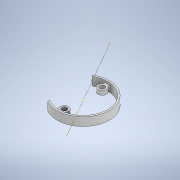
# Autodesk Inventor part: Parachute_Verb
Saved by Autodesk Inventor 2020 (Build 240168000, 168)
## iProperties
Created: 2022-04-20
Part Number: Parachute_Verb
Material: Generisch
Document SubType Name: Modeling
Designer: sp
Density: 1 g/cm^3
Appearance: Vorgabe
Author: sp
Autodesk Inventor part; units mm, degrees
ref_plane "YZ Plane" through (0, 0, 0) normal (1, 0, 0) x (0, 1, 0)
ref_plane "XZ Plane" through (0, 0, 0) normal (0, 1, 0) x (-1, 0, 0)
ref_plane "XY Plane" through (0, 0, 0) normal (0, 0, 1) x (1, 0, 0)
sketch "Skizze1" plane through (0, 0, 0) normal (0, 1, 0) x (-1, 0, 0)
  circle A0 centre (0, 0) radius 29
  circle A1 centre (0, 0) radius 31
  dimension "d0" = 58
  dimension "d1" = 62
  constraints: 2 centre point, 2 coincident
  measures "d0" diameter of A0
  measures "d1" diameter of A1
extrude "Extrusion1" add sketch "Skizze1" along normal mid plane 10
sketch "Skizze2" plane through (0, 0, 0) normal (0, 1, 0) x (-1, 0, 0)
  circle A0 centre (0, 22.5) radius 3
  circle A1 centre (0, -22.5) radius 3
  line L0 (44.9262, 0) -> (-43.1306, 0) construction
  circle A2 centre (0, -22.5) radius 5
  circle A3 centre (0, 22.5) radius 5
  line L1 (0, 38.6377) -> (0, -60.2779) construction
  line L2 (3, 30.0945) -> (-3, 30.0945)
  line L3 (-3, 30.0945) -> (-3, -30.0165)
  line L4 (-3, -30.0165) -> (3, -30.0165)
  line L5 (3, -30.0165) -> (3, 30.0945)
  point P0 (0, 0)
  point P1 (-3, 26.5)
  point P2 (3, 26.5)
  point P3 (-3, -26.5)
  point P4 (3, -26.5)
  dimension "d4" = 45
  dimension "d5" = 6
  dimension "d6" = 6
  dimension "d7" = 10
  dimension "d8" = 10
  dimension "d9" = 6
  constraints: 12 end point, 4 centre point, 2 coincident, 2 horizontal, 2 parallel, 2 point on line, 1 perpendicular, 1 symmetric about line, 1 vertical, 1 other
  measures "d4" distance of A1.centre A0.centre
  measures "d5" diameter of A1
  measures "d6" diameter of A0
  measures "d7" diameter of A3
  measures "d8" diameter of A2
  measures "d9" distance between parallel lines of L3 L5
extrude "Extrusion2" add sketch "Skizze2" along normal mid plane 5 contours L5 A3 L3 A0 | L5 A3 | A0 L3 A3 L5 | L3 A3 | A3 L3 L2 L5 | L5 A1 L3 A2 | A2 L5 | L3 A2 | L5 A2 L3 A1 | A2 L5 L4 L3
sketch "Skizze3" plane through (0, 0, 0) normal (0, 1, 0) x (-1, 0, 0)
  line L0 (-33.7018, 58.3732) -> (42.9469, -74.3862) construction
  line L1 (43.8309, 75.9173) -> (-26.6916, -46.2313) construction
  line L2 (0, 58.0617) -> (0, -82.342) construction
  circle A0 centre (0, 0) radius 31
  circle A1 centre (0, 0) radius 29
  line L3 (17.8979, 31) -> (12.398, 21.474)
  line L4 (13.0797, -22.6548) -> (20.1593, -34.9169)
  point P0 (14.5, -25.1147)
  point P1 (15.5, -26.8468)
  point P2 (15.5, 26.8468)
  point P3 (14.5, 25.1147)
  dimension "d12" = 120
  dimension "d13" = 30
  constraints: 10 end point, 7 point on line, 3 coincident, 2 centre point, 1 vertical
  measures "d12" angle of L0 L1
  measures "d13" angle of L2 L0
extrude "Extrusion3" cut sketch "Skizze3" along normal mid plane 10 contours A0 L4 A1 L3 picked at (30.1075, -2.1484)
sketch "Skizze4" plane through (0, 0, 0) normal (0, 1, 0) x (-1, 0, 0)
  line L0 (-8.0451, 13.9345) -> (38.1422, -66.0642) construction
  line L1 (15.5, -26.8468) -> (14.5, -25.1147) construction
  point P0 (0, 0)
  point P1 (15, -25.9808)
  constraints: 2 end point, 2 point on line, 1 midpoint
